Autodesk Inventor part; units mm, degrees
(part 2 of 2)
  line L319 (-28.6263, 18.3241) -> (-28.6263, 16.0044)
  line L320 (-28.6263, 16.0044) -> (-25.6449, 16.0044)
  line L321 (-25.6449, 18.3241) -> (-28.6263, 18.3241)
  line L322 (-29.7503, 19.4482) -> (-24.5209, 19.4482)
  line L323 (-29.5884, 13.8513) -> (-27.9357, 13.8513)
  line L324 (-29.5884, 12.8808) -> (-29.5884, 13.8513)
  line L325 (-29.7503, 14.8804) -> (-29.7503, 19.4482)
  line L326 (-26.6942, 13.8513) -> (-19.7097, 13.8513)
  line L327 (-23.8, 11.9101) -> (-23.8, 12.8808)
  line L328 (-25.8364, 11.9101) -> (-23.8, 11.9101)
  line L329 (-24.7124, 10.786) -> (-24.7124, 8.4664)
  line L330 (-21.731, 8.4664) -> (-21.731, 10.786)
  line L331 (-24.7124, 8.4664) -> (-21.731, 8.4664)
  line L332 (-21.731, 10.786) -> (-24.7124, 10.786)
  line L333 (-26.6942, 14.8804) -> (-26.6942, 13.8513)
  line L334 (-24.5209, 14.8804) -> (-26.6942, 14.8804)
  line L335 (-20.607, 11.9101) -> (-20.607, 7.3423)
  line L336 (-20.607, 7.3423) -> (-25.8364, 7.3423)
  line L337 (-25.8364, 7.3423) -> (-25.8364, 11.9101)
  line L338 (-27.9357, 14.8804) -> (-29.7503, 14.8804)
  line L339 (-37.8438, 41.8417) -> (-37.8438, 39.522)
  line L340 (-41.854, 38.3672) -> (-47.0835, 38.3672)
  line L341 (-45.9594, 39.4913) -> (-42.9781, 39.4913)
  line L342 (-42.9781, 39.4913) -> (-42.9781, 41.8109)
  line L343 (-39.6887, 44.9654) -> (-33.9003, 44.9654)
  line L344 (-43.779, 42.935) -> (-41.854, 42.935)
  line L345 (-42.9781, 41.8109) -> (-45.9594, 41.8109)
  line L346 (-47.8027, 44.9654) -> (-40.8666, 44.9654)
  line L347 (-43.779, 43.9948) -> (-43.779, 42.935)
  line L348 (-44.8621, 42.935) -> (-44.8621, 43.9948)
  line L349 (-47.0835, 42.935) -> (-44.8621, 42.935)
  line L350 (-44.8621, 43.9948) -> (-47.8027, 43.9948)
  line L351 (-45.9594, 41.8109) -> (-45.9594, 39.4913)
  line L352 (-47.0835, 38.3672) -> (-47.0835, 42.935)
  line L353 (-35.553, 43.9948) -> (-35.553, 42.9657)
  line L354 (-40.8666, 44.9654) -> (-40.8666, 45.9361)
  line L355 (-41.854, 42.935) -> (-41.854, 38.3672)
  line L356 (-40.8666, 45.9361) -> (-42.8818, 45.9361)
  line L357 (-47.8027, 43.9948) -> (-47.8027, 44.9654)
  line L358 (-38.9678, 38.398) -> (-38.9678, 42.9657)
  line L359 (-34.8624, 39.522) -> (-34.8624, 41.8417)
  line L360 (-34.8624, 41.8417) -> (-37.8438, 41.8417)
  line L361 (-37.8438, 39.522) -> (-34.8624, 39.522)
  line L362 (-33.7384, 38.398) -> (-38.9678, 38.398)
  line L363 (-33.9003, 43.9948) -> (-35.553, 43.9948)
  line L364 (-33.9003, 44.9654) -> (-33.9003, 43.9948)
  line L365 (-33.7384, 42.9657) -> (-33.7384, 38.398)
  line L366 (-36.7945, 43.9948) -> (-43.779, 43.9948)
  line L367 (-39.6887, 45.9361) -> (-39.6887, 44.9654)
  line L368 (-37.6523, 45.9361) -> (-39.6887, 45.9361)
  line L369 (-38.7764, 47.0601) -> (-38.7764, 49.3798)
  line L370 (-41.7577, 49.3798) -> (-41.7577, 47.0601)
  line L371 (-38.7764, 49.3798) -> (-41.7577, 49.3798)
  line L372 (-41.7577, 47.0601) -> (-38.7764, 47.0601)
  line L373 (-36.7945, 42.9657) -> (-36.7945, 43.9948)
  line L374 (-38.9678, 42.9657) -> (-36.7945, 42.9657)
  line L375 (-42.8818, 45.9361) -> (-42.8818, 50.5038)
  line L376 (-42.8818, 50.5038) -> (-37.6523, 50.5038)
  line L377 (-37.6523, 50.5038) -> (-37.6523, 45.9361)
  line L378 (-35.553, 42.9657) -> (-33.7384, 42.9657)
  line L379 (-40.5846, 75.534) -> (-40.5846, 13.366) construction
  line L380 (-23.2199, 44.9654) -> (-23.2199, 45.9361)
  line L381 (-23.2199, 45.9361) -> (-25.235, 45.9361)
  line L382 (-19.1478, 43.9948) -> (-26.1323, 43.9948)
  line L383 (-24.111, 47.0601) -> (-21.1296, 47.0601)
  line L384 (-20.0056, 45.9361) -> (-22.042, 45.9361)
  line L385 (-24.111, 49.3798) -> (-24.111, 47.0601)
  line L386 (-25.235, 45.9361) -> (-25.235, 50.5038)
  line L387 (-21.1296, 47.0601) -> (-21.1296, 49.3798)
  line L388 (-21.1296, 49.3798) -> (-24.111, 49.3798)
  line L389 (-25.235, 50.5038) -> (-20.0056, 50.5038)
  line L390 (-20.0056, 50.5038) -> (-20.0056, 45.9361)
  line L391 (-22.042, 45.9361) -> (-22.042, 44.9654)
  line L392 (-24.2073, 38.3672) -> (-29.4368, 38.3672)
  line L393 (-28.3127, 39.4913) -> (-25.3314, 39.4913)
  line L394 (-25.3314, 39.4913) -> (-25.3314, 41.8109)
  line L395 (-26.1323, 42.935) -> (-24.2073, 42.935)
  line L396 (-25.3314, 41.8109) -> (-28.3127, 41.8109)
  line L397 (-30.156, 44.9654) -> (-23.2199, 44.9654)
  line L398 (-27.2154, 42.935) -> (-27.2154, 43.9948)
  line L399 (-30.156, 43.9948) -> (-30.156, 44.9654)
  line L400 (-27.2154, 43.9948) -> (-30.156, 43.9948)
  line L401 (-29.4368, 42.935) -> (-27.2154, 42.935)
  line L402 (-28.3127, 41.8109) -> (-28.3127, 39.4913)
  line L403 (-29.4368, 38.3672) -> (-29.4368, 42.935)
  line L404 (-26.1323, 43.9948) -> (-26.1323, 42.935)
  line L405 (-20.1971, 41.8417) -> (-20.1971, 39.522)
  line L406 (-22.042, 44.9654) -> (-16.2536, 44.9654)
  line L407 (-17.9063, 43.9948) -> (-17.9063, 42.9657)
  line L408 (-24.2073, 42.935) -> (-24.2073, 38.3672)
  line L409 (-21.3211, 38.398) -> (-21.3211, 42.9657)
  line L410 (-21.3211, 42.9657) -> (-19.1478, 42.9657)
  line L411 (-19.1478, 42.9657) -> (-19.1478, 43.9948)
  line L412 (-16.2536, 44.9654) -> (-16.2536, 43.9948)
  line L413 (-16.2536, 43.9948) -> (-17.9063, 43.9948)
  line L414 (-17.2157, 41.8417) -> (-20.1971, 41.8417)
  line L415 (-17.9063, 42.9657) -> (-16.0917, 42.9657)
  line L416 (-20.1971, 39.522) -> (-17.2157, 39.522)
  line L417 (-16.0917, 38.398) -> (-21.3211, 38.398)
  line L418 (-16.0917, 42.9657) -> (-16.0917, 38.398)
  line L419 (-17.2157, 39.522) -> (-17.2157, 41.8417)
  line L420 (-40.5846, 75.534) -> (-22.9266, 44.4801) construction
  line L421 (-40.5734, 44.4801) -> (-22.9154, 75.534) construction
  line L422 (-29.0148, 57.3686) -> (-29.0148, 55.049)
  line L423 (-33.025, 53.8941) -> (-38.2545, 53.8941)
  line L424 (-37.1304, 55.0182) -> (-34.1491, 55.0182)
  line L425 (-34.1491, 55.0182) -> (-34.1491, 57.3379)
  line L426 (-30.8597, 60.4923) -> (-25.0713, 60.4923)
  line L427 (-34.95, 58.4619) -> (-33.025, 58.4619)
  line L428 (-34.1491, 57.3379) -> (-37.1304, 57.3379)
  line L429 (-38.9737, 60.4923) -> (-32.0376, 60.4923)
  line L430 (-34.95, 59.5218) -> (-34.95, 58.4619)
  line L431 (-36.0331, 58.4619) -> (-36.0331, 59.5218)
  line L432 (-38.2545, 58.4619) -> (-36.0331, 58.4619)
  line L433 (-36.0331, 59.5218) -> (-38.9737, 59.5218)
  line L434 (-37.1304, 57.3379) -> (-37.1304, 55.0182)
  line L435 (-38.2545, 53.8941) -> (-38.2545, 58.4619)
  line L436 (-26.724, 59.5218) -> (-26.724, 58.4927)
  line L437 (-32.0376, 60.4923) -> (-32.0376, 61.463)
  line L438 (-33.025, 58.4619) -> (-33.025, 53.8941)
  line L439 (-32.0376, 61.463) -> (-34.0527, 61.463)
  line L440 (-38.9737, 59.5218) -> (-38.9737, 60.4923)
  line L441 (-30.1388, 53.9249) -> (-30.1388, 58.4927)
  line L442 (-26.0334, 55.049) -> (-26.0334, 57.3686)
  line L443 (-26.0334, 57.3686) -> (-29.0148, 57.3686)
  line L444 (-29.0148, 55.049) -> (-26.0334, 55.049)
  line L445 (-24.9094, 53.9249) -> (-30.1388, 53.9249)
  line L446 (-25.0713, 59.5218) -> (-26.724, 59.5218)
  line L447 (-25.0713, 60.4923) -> (-25.0713, 59.5218)
  line L448 (-24.9094, 58.4927) -> (-24.9094, 53.9249)
  line L449 (-27.9655, 59.5218) -> (-34.95, 59.5218)
  line L450 (-30.8597, 61.463) -> (-30.8597, 60.4923)
  line L451 (-28.8233, 61.463) -> (-30.8597, 61.463)
  line L452 (-29.9473, 62.587) -> (-29.9473, 64.9067)
  line L453 (-32.9287, 64.9067) -> (-32.9287, 62.587)
  line L454 (-29.9473, 64.9067) -> (-32.9287, 64.9067)
  line L455 (-32.9287, 62.587) -> (-29.9473, 62.587)
  line L456 (-27.9655, 58.4927) -> (-27.9655, 59.5218)
  line L457 (-30.1388, 58.4927) -> (-27.9655, 58.4927)
  line L458 (-34.0527, 61.463) -> (-34.0527, 66.0308)
  line L459 (-34.0527, 66.0308) -> (-28.8233, 66.0308)
  line L460 (-28.8233, 66.0308) -> (-28.8233, 61.463)
  line L461 (-26.724, 58.4927) -> (-24.9094, 58.4927)
  line L462 (-50.4359, 83.933) -> (-54.8326, 75.2962)
  line L463 (-54.8326, 75.2962) -> (-56.2816, 75.2962)
  line L464 (-56.2816, 75.2962) -> (-51.638, 84.2623)
  line L465 (-51.638, 84.2623) -> (-56.8827, 84.2623)
  line L466 (-56.8827, 84.2623) -> (-56.8827, 85.4562)
  line L467 (-56.8827, 85.4562) -> (-50.4359, 85.4562)
  line L468 (-50.4359, 85.4562) -> (-50.4359, 83.933)
  line L469 (-13.0641, 5.1366) -> (-8.6674, 13.7735)
  line L470 (-8.6674, 13.7735) -> (-7.2184, 13.7735)
  line L471 (-7.2184, 13.7735) -> (-11.862, 4.8073)
  line L472 (-11.862, 4.8073) -> (-6.6173, 4.8073)
  line L473 (-6.6173, 4.8073) -> (-6.6173, 3.6135)
  line L474 (-6.6173, 3.6135) -> (-13.0641, 3.6135)
  line L475 (-13.0641, 3.6135) -> (-13.0641, 5.1366)
  line L476 (-13.0641, 5.1366) -> (-8.6674, 13.7735)
  line L477 (-8.6674, 13.7735) -> (-7.2184, 13.7735)
  line L478 (-7.2184, 13.7735) -> (-11.862, 4.8073)
  line L479 (-11.862, 4.8073) -> (-6.6173, 4.8073)
  line L480 (-6.6173, 4.8073) -> (-6.6173, 3.6135)
  line L481 (-6.6173, 3.6135) -> (-13.0641, 3.6135)
  line L482 (-13.0641, 3.6135) -> (-13.0641, 5.1366)
  line L483 (-50.4359, 83.933) -> (-54.8326, 75.2962)
  line L484 (-54.8326, 75.2962) -> (-56.2816, 75.2962)
  line L485 (-56.2816, 75.2962) -> (-51.638, 84.2623)
  line L486 (-51.638, 84.2623) -> (-56.8827, 84.2623)
  line L487 (-56.8827, 84.2623) -> (-56.8827, 85.4562)
  line L488 (-56.8827, 85.4562) -> (-50.4359, 85.4562)
  line L489 (-50.4359, 85.4562) -> (-50.4359, 83.933)
  point P0 (-53.7479, 68.8958)
  point P1 (-9.7521, 20.0042)
  point P2 (-41.8348, 101.4209)
  point P3 (-53.7479, 68.8958)
  point P4 (-9.7521, 20.0042)
  point P5 (-1, 6.9835)
  point P6 (-94.7005, 61.8998)
  point P7 (-94.7005, 61.8998)
  point P8 (-22.9154, 13.366)
  point P9 (-22.9154, 13.366)
  point P10 (-22.9154, 13.366)
  point P11 (-31.7444, 60.007)
  point P12 (-31.7444, 60.007)
  point P13 (-31.7444, 60.007)
  dimension "d155" = 8.4153
  dimension "d157" = 0.508
  dimension "d158" = 4.5466
  dimension "d159" = 0.508
  dimension "d160" = 4.5466
  constraints: 898 end point, 50 parallel, 20 perpendicular, 14 horizontal, 6 midpoint, 2 symmetric about line, 1 vertical, 14 other
  measures "d155" distance of L174.end L172.start
  measures "d157" distance between parallel lines of L7 L173
  measures "d158" distance from line of point (-1, 6.983) L172
  measures "d159" distance between parallel lines of L6 L168
  measures "d160" distance between parallel lines of L4 L171
extrude "Extrusion20" add sketch "Sketch17" along normal blind 0.4 contours L48 L49 L73 L71 L76 L69 L86 L79 L85 L67 L62 L68 L84 L80 L87 L77 L82 L60 L55 L61 L81 L78 L83 L70 L75 L72 L74 L50 | L88 L89 L113 L111 L116 L109 L126 L119 L125 L107 L102 L108 L124 L120 L127 L117 L122 L100 L95 L101 L121 L118 L123 L110 L115 L112 L114 L90 | L128 L129 L153 L151 L156 L149 L166 L159 L165 L147 L142 L148 L164 L160 L167 L157 L162 L140 L135 L141 L161 L158 L163 L150 L155 L152 L154 L130 | L219 L225 L226 L229 L230 L231 L234 L232 L233 L249 L247 L248 L257 L256 L237 L238 L239 L235 L246 L245 L244 L241 L255 L254 L258 L228 L223 L224 | L260 L272 L269 L268 L270 L277 L266 L274 L276 L295 L296 L297 L288 L287 L263 L284 L283 L273 L298 L285 L282 L278 L294 L293 L286 L267 L264 L275 | L300 L312 L309 L308 L310 L317 L306 L314 L316 L335 L336 L337 L328 L327 L303 L324 L323 L313 L338 L325 L322 L318 L334 L333 L326 L307 L304 L315 | L340 L352 L349 L348 L350 L357 L346 L354 L356 L375 L376 L377 L368 L367 L343 L364 L363 L353 L378 L365 L362 L358 L374 L373 L366 L347 L344 L355 | L380 L381 L386 L389 L390 L384 L391 L406 L412 L413 L407 L415 L418 L417 L409 L410 L411 L382 L404 L395 L408 L392 L403 L401 L398 L400 L399 L397 | L423 L435 L432 L431 L433 L440 L429 L437 L439 L458 L459 L460 L451 L450 L426 L447 L446 L436 L461 L448 L445 L441 L457 L456 L449 L430 L427 L438 | L462 L463 L464 L465 L466 L467 L468 | L469 L470 L471 L472 L473 L474 L475 bodies 2
sketch "Sketch18" plane through (0, 0, -0.2) normal (0, 0, -1) x (-1, 0, 0)
  line L0 (0, 0) -> (-63.5, 0)
  line L1 (-63.5, 0) -> (-63.5, 88.9)
  line L2 (-63.5, 88.9) -> (0, 88.9)
  line L3 (0, 88.9) -> (0, 0)
  constraints: 8 end point, 2 parallel, 1 horizontal, 1 perpendicular
extrude "Extrusion21" add sketch "Sketch18" along normal blind 0.4 bodies 3
fillet "Fillet2" radius 3.175 8 edges at (63.5, 0, 0.2) (63.5, 88.9, 0.2) (0, 0, 0.2) (0, 88.9, 0.2) (63.5, 0, -0.3) (63.5, 88.9, -0.3) (0, 0, -0.3) (0, 88.9, -0.3)
extrude "Extrusion22" cut sketch "Sketch17" along normal blind 0.4 contours L48 L49 L73 L71 L76 L69 L86 L79 L85 L67 L62 L68 L84 L80 L87 L77 L82 L60 L55 L61 L81 L78 L83 L70 L75 L72 L74 L50 | L88 L89 L113 L111 L116 L109 L126 L119 L125 L107 L102 L108 L124 L120 L127 L117 L122 L100 L95 L101 L121 L118 L123 L110 L115 L112 L114 L90 | L128 L129 L153 L151 L156 L149 L166 L159 L165 L147 L142 L148 L164 L160 L167 L157 L162 L140 L135 L141 L161 L158 L163 L150 L155 L152 L154 L130 | L219 L225 L226 L229 L230 L231 L234 L232 L233 L249 L247 L248 L257 L256 L237 L238 L239 L235 L246 L245 L244 L241 L255 L254 L258 L228 L223 L224 | L260 L272 L269 L268 L270 L277 L266 L274 L276 L295 L296 L297 L288 L287 L263 L284 L283 L273 L298 L285 L282 L278 L294 L293 L286 L267 L264 L275 | L300 L312 L309 L308 L310 L317 L306 L314 L316 L335 L336 L337 L328 L327 L303 L324 L323 L313 L338 L325 L322 L318 L334 L333 L326 L307 L304 L315 | L340 L352 L349 L348 L350 L357 L346 L354 L356 L375 L376 L377 L368 L367 L343 L364 L363 L353 L378 L365 L362 L358 L374 L373 L366 L347 L344 L355 | L380 L381 L386 L389 L390 L384 L391 L406 L412 L413 L407 L415 L418 L417 L409 L410 L411 L382 L404 L395 L408 L392 L403 L401 L398 L400 L399 L397 | L423 L435 L432 L431 L433 L440 L429 L437 L439 L458 L459 L460 L451 L450 L426 L447 L446 L436 L461 L448 L445 L441 L457 L456 L449 L430 L427 L438 | L462 L463 L464 L465 L466 L467 L468 | L469 L470 L471 L472 L473 L474 L475 bodies 3
